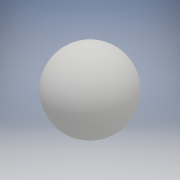
# Autodesk Inventor part: 定位球
Saved by Autodesk Inventor 2017 (Build 210142000, 142)
## iProperties
Part Number: 定位球
Material: 一般
Document SubType Name: Modeling
Designer: Brian
Density: 1 g/cm^3
Appearance: 預設
Author: Brian
Autodesk Inventor part; units mm, degrees
ref_plane "YZ Plane" through (0, 0, 0) normal (1, 0, 0) x (0, 1, 0)
ref_plane "XZ Plane" through (0, 0, 0) normal (0, 1, 0) x (-1, 0, 0)
ref_plane "XY Plane" through (0, 0, 0) normal (0, 0, 1) x (1, 0, 0)
sketch "草圖1" plane through (0, 0, 0) normal (0, 0, 1) x (1, 0, 0)
  circle A0 centre (0, 0) radius 25
  line L0 (0, 25) -> (0, -25)
  dimension "d0" = 50
  dimension "d0" = 50
  constraints: 2 end point, 2 point on circle, 1 centre point, 1 coincident
  measures "d0" diameter of A0
revolve "迴轉1" add sketch "草圖1" angle 360 about axis through (0, 25, 0) along (0, -1, 0) picked at (13.3201, -3.6724) contours A0 L0
